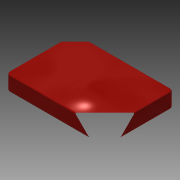
# Autodesk Inventor part: SSD2.5
Saved by Autodesk Inventor 2015 (Build 190159000, 159)
## iProperties
Created: 2016-03-23
Part Number: SSD2.5
Material: Generic
Document SubType Name: Modeling
Designer: Noah
Density: 1 g/cm^3
Appearance: Default
Author: Noah
Autodesk Inventor part; units mm, degrees
ref_plane "YZ Plane" through (0, 0, 0) normal (1, 0, 0) x (0, 1, 0)
ref_plane "XZ Plane" through (0, 0, 0) normal (0, 1, 0) x (-1, 0, 0)
ref_plane "XY Plane" through (0, 0, 0) normal (0, 0, 1) x (1, 0, 0)
sketch "Sketch1" plane through (0, 0, 0) normal (0, 0, 1) x (1, 0, 0)
  line L0 (-50, 35) -> (50, 35)
  line L1 (50, 35) -> (50, -35)
  line L2 (50, -35) -> (-50, -35)
  line L3 (-50, -35) -> (-50, 35)
  point P0 (0, 0)
  dimension "d0" = 100
  dimension "d1" = 70
  dimension "d2" = 35
  dimension "d3" = 50
  constraints: 8 end point, 2 parallel, 1 horizontal, 1 perpendicular
  measures "d0" distance of L1.end L2.end
  measures "d1" distance of L0.end L1.end
  measures "d2" distance from line of L0 point (0, 0)
  measures "d3" distance from line of point (0, 0) L3
extrude "Extrusion1" add sketch "Sketch1" along normal blind 15
fillet "Fillet1" radius 1 8 edges at (50, 0, 15) (0, 35, 15) (0, 35, 0) (50, 0, 0) (-50, 0, 15) (0, -35, 15) (-50, 0, 0) (0, -35, 0)
fillet "Fillet2" radius 4 12 edges at (-49.7071, -34.7071, 14.7071) (-49.7071, -34.7071, 0.2929) (-50, -35, 7.5) (-50, 35, 7.5) (-49.7071, 34.7071, 14.7071) (-49.7071, 34.7071, 0.2929) (50, -35, 7.5) (49.7071, -34.7071, 14.7071) (49.7071, -34.7071, 0.2929) (50, 35, 7.5) (49.7071, 34.7071, 14.7071) (49.7071, 34.7071, 0.2929)
body "Solid1"
